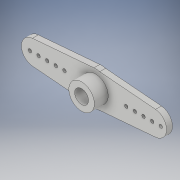
# Autodesk Inventor part: servo arm
Saved by Autodesk Inventor 2017 (Build 210142000, 142)
## iProperties
Created: 2017-02-10
Part Number: servo arm
Material: Generic
Document SubType Name: Modeling
Designer: margr
Density: 1 g/cm^3
Appearance: Default
Author: margr
Autodesk Inventor part; units mm, degrees
ref_plane "YZ Plane" through (0, 0, 0) normal (1, 0, 0) x (0, 1, 0)
ref_plane "XZ Plane" through (0, 0, 0) normal (0, 1, 0) x (-1, 0, 0)
ref_plane "XY Plane" through (0, 0, 0) normal (0, 0, 1) x (1, 0, 0)
sketch "Sketch2" plane through (0, 0, 0) normal (0, 0, 1) x (1, 0, 0)
  line L0 (-10.4096, 0) -> (10.4096, 0) construction
  circle A0 centre (0, 0) radius 6.35
  circle A1 centre (21.7323, 0) radius 4.445
  circle A2 centre (-22.7937, 0) radius 4.445
  line L1 (-23.1652, 4.4294) -> (-0.5307, 6.3278)
  line L2 (22.1038, 4.4294) -> (-0.5307, 6.3278)
  line L3 (22.1038, -4.4294) -> (-0.5307, -6.3278)
  line L4 (-23.1652, -4.4294) -> (-0.5307, -6.3278)
  dimension "d4" = 12.7
  dimension "d5" = 8.89
  dimension "d6" = 8.89
  constraints: 12 end point, 6 point on circle, 6 tangent, 3 centre point, 2 horizontal alignment, 2 parallel, 1 coincident, 1 horizontal, 1 midpoint
  measures "d4" diameter of A0
  measures "d5" diameter of A1
  measures "d6" diameter of A2
extrude "Extrusion2" add sketch "Sketch2" along normal blind 2.159
sketch "Sketch3" plane through (0, 0, 2.159) normal (0, 0, 1) x (1, 0, 0)
  circle A0 centre (0, 0) radius 4.699
  dimension "d11" = 9.398
  constraints: 1 centre point, 1 coincident
  measures "d11" diameter of A0
extrude "Extrusion3" add sketch "Sketch3" along normal blind 5.08
sketch "Sketch4" plane through (0, 0, 7.239) normal (0, 0, 1) x (1, 0, 0)
  circle A0 centre (0, 0) radius 2.54
  dimension "d14" = 5.08
  constraints: 1 centre point, 1 coincident
  measures "d14" diameter of A0
extrude "Extrusion4" cut sketch "Sketch4" against normal through all
sketch "Sketch5" plane through (0, 0, 0) normal (0, 0, -1) x (-1, 0, 0)
  circle A0 centre (24.0637, 0) radius 0.635
  arc A1 (23.1652, -4.4294) -> (23.1652, 4.4294) centre (22.7937, 0) ccw projected
  line L0 (24.0637, 0) -> (4.699, 0)
  circle A2 centre (0, 0) radius 4.699 projected
  circle A3 centre (20.8887, 0) radius 0.635
  circle A4 centre (17.7137, 0) radius 0.635
  circle A5 centre (14.5387, 0) radius 0.635
  circle A6 centre (11.3637, 0) radius 0.635
  line L1 (0, 0) -> (0, -5.8284)
  circle A7 centre (-24.0637, 0) radius 0.635
  circle A8 centre (-20.8887, 0) radius 0.635
  circle A9 centre (-17.7137, 0) radius 0.635
  circle A10 centre (-14.5387, 0) radius 0.635
  circle A11 centre (-11.3637, 0) radius 0.635
  dimension "d17" = 1.27
  dimension "d18" = 2.54
  dimension "d21" = 3.175
  constraints: 10 centre point, 5 symmetric about line, 4 end point, 2 horizontal, 1 horizontal alignment, 1 vertical, 14 other
  measures "d17" diameter of A0
  measures "d21" distance of L0.start A3.centre
extrude "Extrusion5" cut sketch "Sketch5" against normal through all contours A0 | A6 L0 | L0 A6 | A5 L0 | L0 A5 | A4 L0 | L0 A4 | A3 L0 | L0 A3 | A7 | A8 | A9 | A10 | A11
equation "\"d6\" = d5"
body "Solid2"
